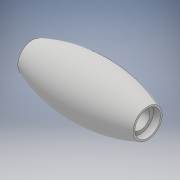
# Autodesk Inventor part: RollerDraft
Saved by Autodesk Inventor 2018 (Build 220112000, 112)
## iProperties
Created: 2017-08-01
Part Number: RollerDraft
Material: Generic
Document SubType Name: Modeling
Designer: P136265
Density: 1 g/cm^3
Appearance: Default
Author: P136265
Autodesk Inventor part; units mm, degrees
ref_plane "YZ Plane" through (0, 0, 0) normal (1, 0, 0) x (0, 1, 0)
ref_plane "XZ Plane" through (0, 0, 0) normal (0, 1, 0) x (-1, 0, 0)
sketch "Sketch1" plane through (0, 0, 0) normal (0, 0, 1) x (1, 0, 0)
  circle A0 centre (0, 0) radius 100 construction
  circle A1 centre (0, 0) radius 75 construction
  circle A2 centre (0, 75) radius 25 construction
  circle A3 centre (0, 0) radius 89 construction
  dimension "d8" = 150
  dimension "d7" = 200
  dimension "d9" = 50
  dimension "d10" = 14
  constraints: 3 centre point, 2 coincident, 2 vertical alignment, 2 other
  measures "d7" diameter of A0
  measures "d9" diameter of A2
sketch "Sketch6" plane through (0, 0, 0) normal (0, 0, 1) x (1, 0, 0)
  point P0 (0, 0)
ref_plane "Work Plane3" through (0, 0, 0) normal (0, -0.7071068, 0.7071068) x (1, 0, 0)
sketch "2d Roller Ellipse" plane through (0, 0, 0) normal (0, -0.7071068, 0.7071068) x (1, 0, 0)
  ellipse E0 centre (0, 0) end of major axis (100, 0) minor radius 70.7107 construction
  ellipse E1 centre (0, 53.033) end of major axis (25, 53.033) minor radius 17.6777 construction
  ellipse E2 centre (0, 0) end of major axis (100, 0) minor radius 70.7107 construction
  circle A0 centre (0, 45.7107) radius 22 construction
  circle A1 centre (0, 45.7107) radius 12.5 construction
  line L0 (0, 58.2107) -> (49.548, 58.2107) construction
  line L1 (49.548, 58.2107) -> (49.548, 45.7107)
  line L2 (0, 58.2107) -> (-49.548, 58.2107) construction
  line L3 (-49.548, 58.2107) -> (-49.548, 45.7107)
  line L4 (0, 45.7107) -> (-49.548, 45.7107)
  ellipse E3 centre (0, 0) end of major axis (97, 0) minor radius 67.7107 (49.548, 58.2107) -> (-49.548, 58.2107) ccw
  line L5 (0, 45.7107) -> (49.548, 45.7107)
  spline S0 degree 5 poles (125, 0) (124.9996, 8.8962) (123.6824, 17.7961) (121.0383, 26.425) (113.3824, 42.8537) (101.833, 56.8343) (95.2127, 63.1614) (80.4494, 74.6213) (63.7738, 83.0792) (54.8985, 86.6443) (36.372, 92.4116) (17.1764, 95.263) (7.3437, 95.9828) (-12.2502, 95.9826) (-31.6302, 93.1025) (-41.1422, 90.9507) (-59.3601, 85.2856) (-76.3656, 76.6479) (-84.2872, 71.6905) (-98.7984, 60.4396) (-110.4889, 46.2955) (-115.3769, 38.6773) (-122.9533, 22.3258) (-125.6666, 4.5154) (-125.6666, -4.5154) (-122.9533, -22.3258) (-115.3769, -38.6773) (-110.4889, -46.2955) (-98.7984, -60.4396) (-84.2872, -71.6905) (-76.3656, -76.6479) (-59.3601, -85.2856) (-41.1422, -90.9507) (-31.6302, -93.1025) (-12.2502, -95.9826) (7.3437, -95.9828) (17.1764, -95.263) (36.372, -92.4116) (54.8985, -86.6443) (63.7738, -83.0792) (80.4494, -74.6213) (95.2127, -63.1614) (101.833, -56.8343) (113.3824, -42.8537) (121.0383, -26.425) (123.6824, -17.7961) (124.9996, -8.8962) (125, 0) knots 0 0 0 0 0 0 0.063791 0.063791 0.063791 0.128941 0.128941 0.128941 0.197218 0.197218 0.197218 0.267663 0.267663 0.267663 0.337325 0.337325 0.337325 0.403955 0.403955 0.403955 0.468142 0.468142 0.468142 0.531858 0.531858 0.531858 0.596045 0.596045 0.596045 0.662675 0.662675 0.662675 0.732337 0.732337 0.732337 0.802782 0.802782 0.802782 0.871059 0.871059 0.871059 0.936209 0.936209 0.936209 1 1 1 1 1 1 construction
  dimension "d53" = 25
  dimension "d55" = 25
  dimension "d61" = 100
  dimension "d62" = 97
  dimension "d63" = 70.7107
  dimension "d64" = 67.7107
  dimension "d54" = 44
  dimension "d59" = 12.5
  dimension "d60" = 12.5
  constraints: 12 end point, 6 horizontal, 2 coincident, 1 centre point, 1 parallel, 1 vertical alignment, 13 other
  measures "d54" diameter of A0
  measures "d59" distance of L0.end L1.end
  measures "d60" distance of L2.end L3.end
revolve "Revolution4" add sketch "2d Roller Ellipse" angle 360 about axis through (0, 32.3223, 32.3223) along (-1, 0, 0)
sketch "Sketch8" plane through (49.548, 32.3223, 32.3223) normal (1, 0, 0) x (0, 0, -1)
  circle A0 centre (0, 0) radius 8
  point P0 (32.3223, -32.3223)
  dimension "d66" = 16
  constraints: 1 centre point
  measures "d66" diameter of A0
extrude "Bore" cut sketch "Sketch8" against normal blind 100
sketch "Sketch9" plane through (49.548, 32.3223, 32.3223) normal (1, 0, 0) x (0, 0, -1)
  circle A0 centre (0, 0) radius 11
  point P0 (32.3223, -32.3223)
  dimension "d71" = 22
  constraints: 1 centre point
  measures "d71" diameter of A0
extrude "Bearing_Area_A" cut sketch "Sketch9" against normal blind 6
sketch "Sketch10" plane through (-49.548, 32.3223, 32.3223) normal (-1, 0, 0) x (0, 0, 1)
  circle A0 centre (0, 0) radius 11
  point P0 (-32.3223, -32.3223)
  dimension "d74" = 22
  constraints: 1 centre point
  measures "d74" diameter of A0
extrude "Bearing_Area_B" cut sketch "Sketch10" against normal blind 6
